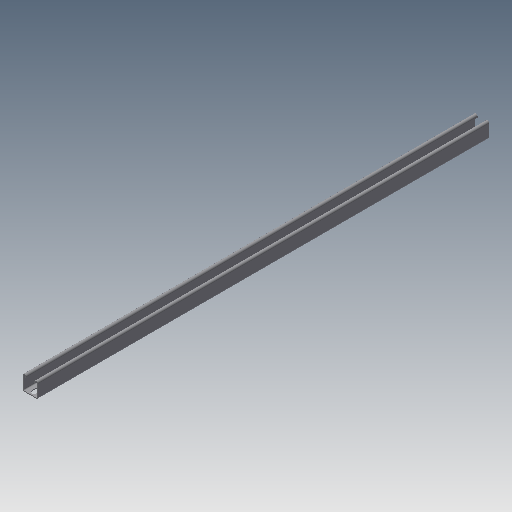
# Autodesk Inventor part: P1000 x 1000
Saved by Autodesk Inventor 2020 (Build 240152000, 152)
## iProperties
Created: 2009-08-10
Part Number: P1000 x 1000
Document SubType Name: Modeling
Designer: Demir Ali
Density: 1 g/cm^3
Description: Unistrut
Material: Generic
Stock Number: NA
Appearance: Default
Mass: 379.032 g
Surface Area: 3142.12 cm^2
Volume: 379.032 cm^3
Title: Purchased Part
Author: Demir Ali
Revision Number: A
Autodesk Inventor part; units mm, degrees
ref_plane "YZ Plane" through (0, 0, 0) normal (1, 0, 0) x (0, 1, 0)
ref_plane "XZ Plane" through (0, 0, 0) normal (0, 1, 0) x (-1, 0, 0)
ref_plane "XY Plane" through (0, 0, 0) normal (0, 0, 1) x (1, 0, 0)
sketch "Sketch1" plane through (0, 0, 0) normal (0, 0, 1) x (1, 0, 0)
  line L0 (20.5, 15.5) -> (20.5, -15.5)
  line L1 (15.5, -20.5) -> (-15.5, -20.5)
  line L2 (-20.5, -15.5) -> (-20.5, 15.5)
  arc A0 (-10.5, 15.5) -> (-20.5, 15.5) centre (-15.5, 15.5) ccw
  arc A1 (20.5, 15.5) -> (10.5, 15.5) centre (15.5, 15.5) ccw
  arc A2 (-20.5, -15.5) -> (-15.5, -20.5) centre (-15.5, -15.5) ccw
  arc A3 (15.5, -20.5) -> (20.5, -15.5) centre (15.5, -15.5) ccw
  line L3 (-10.5, 15.5) -> (-10.5, 13)
  line L4 (-10.5, 13) -> (10.5, 13)
  line L5 (10.5, 13) -> (10.5, 15.5)
  point P0 (0, 0)
  point P1 (20.5, -20.5)
  point P2 (-20.5, -20.5)
  point P3 (-20.5, 0)
  point P4 (0, -20.5)
  dimension "d1" = 41
  dimension "d2" = 41
  dimension "d3" = 5
  dimension "d7" = 5
  dimension "d8" = 2.5
  constraints: 12 end point, 8 point on circle, 8 tangent, 4 centre point, 4 parallel, 4 point on line, 3 horizontal alignment, 2 equal radius, 2 midpoint, 1 horizontal, 1 perpendicular, 1 vertical, 1 vertical alignment
  measures "d1" distance of point (20.5, -20.5) point (-20.5, -20.5)
  measures "d3" radius of A0
  measures "d7" radius of A2
  measures "d8" distance of L3.start L3.end
extrude "Extrusion1" add sketch "Sketch1" along normal blind 1200
shell "Shell1" thickness 2.5 removed faces 3 at (3.5, -9.3333, 1200) at (3.5, -9.3333, 0) at (3.5, 13, 400)
sketch "Sketch2" plane through (-15.5, -20.5, 0) normal (0, -1, 0) x (1, 0, 0)
  line L0 (0, 0) -> (31, 0) projected
  line L1 (8.5, 25) -> (8.5, 39)
  arc A0 (22.5, 39) -> (8.5, 39) centre (15.5, 39) ccw
  line L2 (22.5, 39) -> (22.5, 25)
  arc A1 (8.5, 25) -> (22.5, 25) centre (15.5, 25) ccw
  point P0 (15.5, 0)
  point P1 (15.5, 0)
  dimension "d9" = 7
  dimension "d11" = 25
  dimension "d17" = 28
  constraints: 4 end point, 4 point on circle, 4 tangent, 2 centre point, 2 midpoint, 2 vertical alignment, 1 equal radius, 1 vertical
  measures "d9" radius of A1
  measures "d11" distance from line of L0 A1.centre
extrude "Extrusion2" cut sketch "Sketch2" against normal through all
pattern_linear "Rectangular Pattern1" count 24 spacing 50 along (0, 0, 1) of "Extrusion2"
equation "\"d2\" = d1"
body "Solid1"
